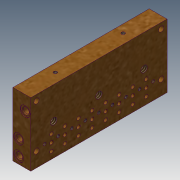
# Autodesk Inventor part: J005162
Saved by Autodesk Inventor 2015 SP1 (Build 190203100, 203)
## iProperties
Created: 2015-04-08
Material: PEEK 1000
Vendor: HHMI: JRC - ID&F
Document SubType Name: Modeling
Designer: JORDANJ
Density: 1.31 g/cm^3
Appearance: Tan
Project: P-171601
Part Number: J005162
Description: COMPONENT OF AN AUTOMATED LIQUID HANDLING MACHINE SPECIFICALLY DESIGNED FOR THE IN SITU RNA HYBRIDIZATION OF DROSOPHILA EMBRYOS
RuleStatus: InUse
AfterDocSave0: file://Part Number Cleaner
LAB/DEPT: STERN (LAB)
REQUESTING SCIENTIST: STERN, DAVID
SURFACE ROUGHNESS: 16 Ra
DESIGN DEPARTMENT: HHMI: JRC - ID&F
SPECIAL FINISH: N/A
ALTERED ITEM PART NUMBER: N/A
ALTERED ITEM VENDOR: N/A
ALTERED ITEM DESCRIPTION: N/A
valve_spacing: 0.3000 in
no_valves: 8.0000 ul
Author: JORDANJ
Revision Number: A
Autodesk Inventor part; units mm, degrees
ref_plane "YZ Plane" through (0, 0, 0) normal (1, 0, 0) x (0, 1, 0)
ref_plane "XZ Plane" through (0, 0, 0) normal (0, 1, 0) x (-1, 0, 0)
ref_plane "XY Plane" through (0, 0, 0) normal (0, 0, 1) x (1, 0, 0)
sketch "Sketch1" plane through (0, 0, 0) normal (0, 0, 1) x (1, 0, 0)
  line L0 (9.9949, 17.907) -> (0, 17.907)
  line L1 (0, 17.907) -> (0, -17.907)
  line L2 (0, -17.907) -> (9.9949, -17.907)
  line L3 (9.9949, -17.907) -> (9.9949, 17.907)
  line L4 (3.175, -4.4958) -> (9.9949, -4.4958)
  line L5 (9.9949, -4.4958) -> (9.9949, -6.477)
  line L6 (9.9949, -6.477) -> (3.175, -6.477)
  line L7 (3.175, -6.477) -> (3.175, -4.4958) construction
  line L8 (0.75, -8.7376) -> (9.9949, -8.7376)
  line L9 (9.9949, -8.7376) -> (9.9949, -10.7188)
  line L10 (9.9949, -10.7188) -> (0.75, -10.7188)
  line L11 (0.75, -10.7188) -> (0.75, -8.7376) construction
  line L12 (3.175, -12.9794) -> (9.9949, -12.9794)
  line L13 (9.9949, -12.9794) -> (9.9949, -14.9606)
  line L14 (9.9949, -14.9606) -> (3.175, -14.9606)
  line L15 (3.175, -14.9606) -> (3.175, -12.9794) construction
  line L16 (2.5798, -5.4864) -> (9.9949, -5.4864)
  line L17 (0.1548, -9.7282) -> (9.9949, -9.7282)
  line L18 (2.5798, -13.97) -> (9.9949, -13.97)
  line L19 (5.6958, -7.4168) -> (9.9949, -7.4168)
  line L20 (9.9949, -7.4168) -> (9.9949, -9.6012)
  line L21 (9.9949, -9.6012) -> (5.6958, -9.6012)
  line L22 (5.6958, -9.6012) -> (5.6958, -7.4168) construction
  line L23 (5.6958, -7.4168) -> (5.0395, -8.509)
  line L24 (5.0395, -8.509) -> (5.6958, -9.6012)
  line L25 (5.0395, -8.509) -> (9.9949, -8.509)
  line L26 (9.9949, 17.145) -> (17.6149, 17.145) construction
  line L27 (17.6149, 17.145) -> (17.6149, -8.509) construction
  line L28 (17.6149, -8.509) -> (9.9949, -8.509) construction
  line L29 (9.9949, -8.509) -> (9.9949, 17.145) construction
  line L30 (3.175, -4.4958) -> (2.5798, -5.4864)
  line L31 (2.5798, -5.4864) -> (3.175, -6.477)
  line L32 (0.75, -8.7376) -> (0.1548, -9.7282)
  line L33 (0.1548, -9.7282) -> (0.75, -10.7188)
  line L34 (3.175, -12.9794) -> (2.5798, -13.97)
  line L35 (2.5798, -13.97) -> (3.175, -14.9606)
  circle A0 centre (3.175, -5.4864) radius 1.1811
  line L36 (4.0069, -13.97) -> (5.9881, -13.97) construction
  line L37 (5.9881, -13.97) -> (5.9881, -17.907) construction
  line L38 (5.9881, -17.907) -> (4.0069, -17.907) construction
  line L39 (4.0069, -17.907) -> (4.0069, -13.97) construction
  line L40 (4.0069, -13.97) -> (4.9975, -13.3748) construction
  line L41 (4.9975, -13.3748) -> (5.9881, -13.97) construction
  line L42 (4.9975, -13.3748) -> (4.9975, -17.907) construction
  circle A1 centre (3.175, -5.4864) radius 3.175 construction
  line L43 (0, -7.2282) -> (0.75, -7.2282)
  line L44 (0.75, -7.2282) -> (0.75, -12.2282)
  line L45 (0.75, -12.2282) -> (0, -12.2282)
  line L46 (0, -12.2282) -> (0, -7.2282)
  line L47 (0, -9.7282) -> (0.75, -9.7282)
  circle A2 centre (0.25, -11.7282) radius 0.5
  line L48 (-6.35, 19.431) -> (17.6149, 19.431)
  line L49 (17.6149, 19.431) -> (17.6149, 17.907)
  line L50 (17.6149, 17.907) -> (-6.35, 17.907)
  line L51 (-6.35, 17.907) -> (-6.35, 19.431)
  line L52 (-6.35, 17.907) -> (0, 17.907)
  line L53 (0, 17.907) -> (0, -17.907)
  line L54 (0, -17.907) -> (-6.35, -17.907)
  line L55 (-6.35, -17.907) -> (-6.35, 17.907)
  line L56 (-12.7, -10.9093) -> (0, -10.9093)
  line L57 (0, -10.9093) -> (0, -11.3093)
  line L58 (0, -11.3093) -> (-12.7, -11.3093)
  line L59 (-12.7, -11.3093) -> (-12.7, -10.9093)
  line L60 (-12.7, -8.5471) -> (0, -8.5471)
  line L61 (0, -8.5471) -> (0, -8.1471)
  line L62 (0, -8.1471) -> (-12.7, -8.1471)
  line L63 (-12.7, -8.1471) -> (-12.7, -8.5471)
  line L64 (-12.7, 8.5471) -> (0, 8.5471)
  line L65 (0, 8.5471) -> (0, 8.1471)
  line L66 (0, 8.1471) -> (-12.7, 8.1471)
  line L67 (-12.7, 8.1471) -> (-12.7, 8.5471)
  line L68 (-12.7, 9.7282) -> (0, 9.7282)
  line L69 (-12.7, 10.9093) -> (0, 10.9093)
  line L70 (0, 10.9093) -> (0, 11.3093)
  line L71 (0, 11.3093) -> (-12.7, 11.3093)
  line L72 (-12.7, 11.3093) -> (-12.7, 10.9093)
  circle A3 centre (6.8199, 9.7282) radius 1.1811
  line L73 (0, 12.5857) -> (0.75, 12.5857)
  line L74 (0.75, 12.5857) -> (0.75, 11.7411)
  line L75 (0.75, 11.7411) -> (5.6104, 11.7412)
  line L76 (5.6104, 11.7412) -> (6.8199, 9.7282)
  line L77 (6.8199, 9.7282) -> (0, 9.7282)
  line L78 (0, 6.8707) -> (0.75, 6.8707)
  line L79 (0.75, 6.8707) -> (0.75, 7.7153)
  line L80 (0.75, 7.7153) -> (5.6104, 7.7152)
  line L81 (5.6104, 7.7152) -> (6.8199, 9.7282)
  line L82 (0, 12.5857) -> (0, 6.8707)
  line L83 (-6.35, 0) -> (9.9949, 0) construction
  line L84 (-12.7, -8.5471) -> (-12.7, -10.9093)
  line L85 (-12.7, 10.9093) -> (-12.7, 8.5471)
  line L86 (0, 10.9093) -> (0, 8.5471)
  line L87 (0, -8.5471) -> (0, -10.9093)
  line L88 (-12.7, -9.7282) -> (0, -9.7282)
  circle A4 centre (6.8199, 9.7282) radius 3.175 construction
  circle A5 centre (6.8199, 9.7282) radius 1.5812 construction
  circle A6 centre (3.175, -13.97) radius 1.1811
  line L89 (3.9053, 19.431) -> (6.0896, 19.431)
  line L90 (6.0896, 19.431) -> (6.0896, 13.7614)
  line L91 (6.0896, 13.7614) -> (3.9053, 13.7614) construction
  line L92 (3.9053, 13.7614) -> (3.9053, 19.431)
  line L93 (3.9053, 13.7614) -> (4.9975, 13.1051)
  line L94 (4.9975, 13.1051) -> (6.0896, 13.7614)
  line L95 (2.9147, 20.5994) -> (7.0803, 20.5994)
  line L96 (7.0803, 20.5994) -> (7.0803, 19.431)
  line L97 (7.0803, 19.431) -> (2.9147, 19.431)
  line L98 (2.9147, 19.431) -> (2.9147, 20.5994)
  line L99 (4.9974, 19.431) -> (4.9975, 13.1051)
  line L100 (4.9975, 20.5994) -> (4.9974, 19.431)
  line L101 (3.9053, 14.6685) -> (6.0896, 14.6685)
  line L102 (-3.5011, 2.413) -> (6.35, 2.413)
  line L103 (6.35, 2.413) -> (6.35, -2.413) construction
  line L104 (6.35, -2.413) -> (-3.5011, -2.413)
  line L105 (-3.5011, -2.413) -> (-3.5011, 2.413) construction
  line L106 (6.35, 2.413) -> (7.7999, 0)
  line L107 (7.7999, 0) -> (6.35, -2.413)
  line L108 (-3.5011, 2.413) -> (-6.35, 4.8895)
  line L109 (-6.35, 4.8895) -> (-6.35, -4.8895)
  line L110 (-6.35, -4.8895) -> (-3.5011, -2.413)
  line L111 (-6.35, 0) -> (7.7999, 0)
  line L112 (5.2917, 2.413) -> (5.2917, -2.413) construction
  circle A7 centre (6.8199, 9.7282) radius 1.5
  circle A8 centre (6.8199, 9.7282) radius 2.5
  circle A9 centre (3.175, -5.4864) radius 1.5
  circle A10 centre (3.175, -5.4864) radius 2.5
  circle A11 centre (3.175, -13.97) radius 1.5
  circle A12 centre (3.175, -13.97) radius 2.5
  point P0 (0, 0)
  point P1 (4.9975, 17.907)
  point P2 (0, 0)
  dimension "d2" = 118
  dimension "d3" = 2.1844
  dimension "d4" = 1.9812
  dimension "d5" = 5.461
  dimension "d6" = 1.2192
  dimension "d7" = 3.0226
  dimension "d8" = 4.2992
  dimension "d9" = 118
  dimension "d10" = 7.62
  dimension "d11" = 25.654
  dimension "d12" = 0.762
  dimension "d14" = 2.3622
  dimension "d15" = 2.9464
  dimension "d17" = 1
  dimension "d20" = 3
  dimension "d21" = 1.524
  dimension "d22" = 9.398
  dimension "d26" = 6.35
  dimension "port_depth" = 6.35
  dimension "d29" = 118
  dimension "d30" = 4.0259
  dimension "d32" = 5.715
  dimension "d35" = 0.75
  dimension "d36" = 8.1788
  dimension "d38" = 9.9949
  dimension "d45" = 6.35
  dimension "port_id" = 2.3622
  dimension "port_od" = 3.1623
  dimension "d101" = 8.1788
  dimension "d102" = 3.1623
  dimension "d104" = 5.6388
  dimension "d107" = 3.1623
  dimension "d134" = 118
  dimension "d137" = 2.1844
  dimension "d138" = 1.1684
  dimension "d139" = 4.1656
  dimension "drilldepth" = 4.1456
  dimension "d158" = 4.7625
  dimension "d159" = 0.9071
  dimension "threaddepth" = 3.2385
  dimension "d161" = 118
  dimension "d162" = 82
  dimension "d163" = 9.779
  dimension "d164" = 4.826
  dimension "d165" = 12.7
  dimension "d166" = 5.2917
  dimension "d183" = 0.25
  dimension "d212" = 1
  dimension "d213" = 3
  dimension "d284" = 6.35
  dimension "d296" = 0.75
  constraints: 226 end point, 33 parallel, 27 collinear, 22 horizontal, 22 midpoint, 15 perpendicular, 13 equal length, 12 centre point, 12 vertical, 8 coincident, 8 symmetric about line, 6 equal radius, 5 point on line, 3 tangent, 1 vertical alignment, 9 other
  measures "d2" angle of L24 L23
  measures "d3" distance between parallel lines of L21 L19
  measures "d4" distance between parallel lines of L14 L12
  measures "d5" distance between parallel lines of L25 L18
  measures "d6" distance between parallel lines of L17 L25
  measures "d7" distance between parallel lines of L16 L25
  measures "d8" distance of L19.start L19.end
  measures "d9" angle of L41 L40
  measures "d10" distance of L26.start L26.end
  measures "d11" distance of L26.end L27.end
  measures "d12" distance between parallel lines of L26 L0
  measures "d14" diameter of A0
  measures "d15" distance between parallel lines of L38 L14
  measures "d17" diameter of A2
  measures "d21" distance of L48.end L49.end
  measures "d22" distance between parallel lines of L2 L28
  measures "d26" distance between parallel lines of L55 L59
  measures "port_depth" distance between parallel lines of L57 L55
  measures "d29" angle of L81 L76
  measures "d30" distance between parallel lines of L80 L75
  measures "d32" distance of L73.start L78.start
  measures "d35" distance between parallel lines of L82 L79
  measures "d36" distance between parallel lines of L52 L68
  measures "d38" distance of L1.end L2.end
  measures "d45" distance of L53.end L54.end
  measures "port_id" distance between parallel lines of L60 L56
  measures "port_od" distance between parallel lines of L58 L62
  measures "d101" distance between parallel lines of L54 L88
  measures "d102" distance between parallel lines of L71 L66
  measures "d104" distance edge to line of A3 L82
  measures "d107" diameter of A5
  measures "d134" angle of L94 L93
  measures "d137" distance between parallel lines of L90 L92
  measures "d138" distance of L97.end L95.start
  measures "d139" distance between parallel lines of L96 L98
  measures "drilldepth" distance between parallel lines of L91 L0
  measures "d158" distance between parallel lines of L97 L101
  measures "d159" distance between parallel lines of L101 L91
  measures "threaddepth" distance between parallel lines of L101 L0
  measures "d161" angle of L107 L106
  measures "d162" angle of L110 L108
  measures "d163" distance of L108.end L109.end
  measures "d164" distance between parallel lines of L104 L102
  measures "d165" distance between parallel lines of L103 L109
  measures "d166" distance between parallel lines of L112 L1
  measures "d183" distance centre to line of A2 L1
  measures "d212" radial gap between concentric circles of A8 A7
  measures "d213" diameter of A7
  measures "d284" diameter of A4
  measures "d296" distance of L44.end L45.end
sketch "Sketch2" plane through (0, 0, 0) normal (1, 0, 0) x (0, 1, 0)
  line L0 (17.907, 11.6205) -> (-17.907, 11.6205)
  line L1 (-17.907, 11.6205) -> (-17.907, -64.9605)
  line L2 (-17.907, -64.9605) -> (17.907, -64.9605)
  line L3 (17.907, -64.9605) -> (17.907, 11.6205)
  circle A0 centre (-13.97, 0) radius 0.9906 construction
  circle A1 centre (-9.7282, 0) radius 0.9906 construction
  circle A2 centre (-5.4864, 0) radius 1.5812 construction
  line L4 (-8.509, 3.81) -> (-8.509, -3.81) construction
  circle A3 centre (9.7282, 0) radius 1.5812 construction
  circle A4 centre (-8.509, -3.81) radius 2.3876 construction
  circle A5 centre (-8.509, 3.81) radius 2.3876 construction
  line L5 (17.145, 3.81) -> (-17.907, 3.81) construction
  line L6 (-17.907, 3.81) -> (-17.907, -3.81) construction
  line L7 (-17.907, -3.81) -> (17.145, -3.81) construction
  line L8 (17.145, -3.81) -> (17.145, 3.81) construction
  line L9 (17.145, 0) -> (-17.907, 0) construction
  line L10 (24.257, 1.5875) -> (17.145, 1.5875) construction
  line L11 (17.145, 1.5875) -> (17.145, 0.9525) construction
  line L12 (17.145, 0.9525) -> (24.257, 0.9525) construction
  line L13 (24.257, 0.9525) -> (24.257, 1.5875) construction
  line L14 (24.257, -1.5875) -> (17.145, -1.5875) construction
  line L15 (17.145, -1.5875) -> (17.145, -0.9525) construction
  line L16 (17.145, -0.9525) -> (24.257, -0.9525) construction
  line L17 (24.257, -0.9525) -> (24.257, -1.5875) construction
  line L18 (24.257, 1.27) -> (17.145, 1.27) construction
  line L19 (24.257, -1.27) -> (17.145, -1.27) construction
  line L20 (17.907, -26.67) -> (-17.907, -26.67) construction
  line L21 (-8.509, -3.81) -> (-8.509, -11.43) construction
  circle A6 centre (-8.509, -11.43) radius 2.3876 construction
  line L22 (-8.509, -11.43) -> (-8.509, -19.05) construction
  circle A7 centre (-8.509, -19.05) radius 2.3876 construction
  line L23 (-8.509, -19.05) -> (-8.509, -26.67) construction
  circle A8 centre (-8.509, -26.67) radius 2.3876 construction
  line L24 (-8.509, -26.67) -> (-8.509, -34.29) construction
  circle A9 centre (-8.509, -34.29) radius 2.3876 construction
  line L25 (-8.509, -34.29) -> (-8.509, -41.91) construction
  circle A10 centre (-8.509, -41.91) radius 2.3876 construction
  line L26 (-8.509, -41.91) -> (-8.509, -49.53) construction
  circle A11 centre (-8.509, -49.53) radius 2.3876 construction
  line L27 (-8.509, -49.53) -> (-8.509, -57.15) construction
  circle A12 centre (-8.509, -57.15) radius 2.3876 construction
  circle A13 centre (14.6685, 8.382) radius 1.4224
  circle A14 centre (-9.7282, 8.382) radius 1.4224
  circle A15 centre (14.6685, 8.382) radius 2.8575
  circle A16 centre (14.6685, 8.382) radius 3.2385 construction
  line L28 (0, -64.9605) -> (0, 11.6205) construction
  circle A17 centre (14.6685, -61.722) radius 1.4224
  circle A18 centre (-9.7282, -61.722) radius 1.4224
  line L29 (-9.7282, 6.1976) -> (14.6685, 6.1976)
  line L30 (16.8529, 8.382) -> (16.8529, 14.859)
  line L31 (14.6685, 17.0434) -> (-9.7282, 17.0434)
  line L32 (-11.9126, 14.859) -> (-11.9126, 8.382)
  arc A19 (-11.9126, 8.382) -> (-9.7282, 6.1976) centre (-9.7282, 8.382) ccw
  arc A20 (-9.7282, 17.0434) -> (-11.9126, 14.859) centre (-9.7282, 14.859) ccw
  arc A21 (16.8529, 14.859) -> (14.6685, 17.0434) centre (14.6685, 14.859) ccw
  arc A22 (14.6685, 6.1976) -> (16.8529, 8.382) centre (14.6685, 8.382) ccw
  circle A23 centre (14.6685, 14.859) radius 1.4224
  circle A24 centre (-9.7282, 14.859) radius 1.4224
  point P0 (0, 0)
  point P1 (-9.7282, 0)
  point P2 (-8.509, 0)
  point P3 (-8.509, 0)
  point P4 (-8.509, 0)
  point P5 (-13.97, 0)
  point P6 (-13.97, 0)
  point P7 (-13.97, 0)
  point P8 (17.907, 0)
  point P9 (17.907, 0)
  point P10 (17.907, 0)
  point P11 (-8.509, 0)
  point P12 (-8.509, -7.62)
  point P13 (-8.509, -15.24)
  point P14 (-8.509, -22.86)
  point P15 (-8.509, -30.48)
  point P16 (-8.509, -38.1)
  point P17 (-8.509, -45.72)
  point P18 (-8.509, -53.34)
  point P19 (-11.9126, 11.6205)
  dimension "d44" = 1.9812
  dimension "valve_spacing" = 7.62
  dimension "d48" = 4.7752
  dimension "d49" = 7.62
  dimension "d51" = 25.654
  dimension "d52" = 0.635
  dimension "d53" = 2.54
  dimension "d54" = 32.766
  dimension "d57" = 7.62
  dimension "d62" = 30.48
  dimension "d103" = 3.1623
  dimension "d245" = 2.8448
  dimension "d249" = 5.715
  dimension "d272" = 24.3967
  dimension "d273" = 0.381
  dimension "d283" = 0.762
  dimension "d293" = 70.104
  dimension "d294" = 24.3967
  dimension "d295" = 76.581
  constraints: 67 end point, 25 centre point, 14 coincident, 12 midpoint, 11 tangent, 8 equal radius, 8 parallel, 8 point on circle, 8 symmetric about line, 4 horizontal, 4 perpendicular, 4 point on line, 3 collinear, 3 vertical, 2 concentric, 1 horizontal alignment, 1 vertical alignment, 44 other
  measures "d44" diameter of A0
  measures "valve_spacing" distance of L4.start L4.end
  measures "d48" diameter of A4
  measures "d49" distance of L5.end L6.end
  measures "d51" distance between parallel lines of L8 L4
  measures "d52" distance between parallel lines of L12 L10
  measures "d53" distance between parallel lines of L19 L18
  measures "d54" distance between parallel lines of L13 L4
  measures "d57" distance of L4.start L21.start
  measures "d62" distance from line of L20 A5.centre
  measures "d103" diameter of A2
  measures "d245" diameter of A13
  measures "d249" diameter of A15
  measures "d272" distance of A14.centre A13.centre
  measures "d273" radial gap between concentric circles of A16 A15
  measures "d283" radial gap between concentric circles of A22 A13
  measures "d293" distance of A17.centre A13.centre
  measures "d294" distance of A18.centre A17.centre
  measures "d295" distance of A17.centre A23.centre
extrude "Extrusion1" add sketch "Sketch2" along normal blind 9.9949 contours L3 L2 L1 L0 L32 A19 L29 A15 L30 | L30 A15 L29 A19 L32 L0 | L30 A22 L29 A15 | A15 L29 A22 L30
extrude "Extrusion2" add sketch "Sketch2" against normal blind 6.35 separate body contours L3 L2 L1 L0 L32 A19 L29 A15 L30 | L30 A15 L29 A19 L32 L0 | L30 A22 L29 A15 | A15 L29 A22 L30
revolve "Revolution3" cut sketch "Sketch1" angle 360 about axis through (2.5798, -13.97, 0) along (1, 0, 0) bodies 2 1 contours L3 L14 A12 L18 | A12 L14 A11 L18 | A11 L14 A6 L18 | A6 L14 L35 L18
revolve "Revolution4" cut sketch "Sketch1" angle 360 about axis through (0.1548, -9.7282, 0) along (1, 0, 0) bodies 1 contours L3 L10 L44 L17 | L44 L33 L17
revolve "Revolution5" cut sketch "Sketch1" angle 360 about axis through (2.5798, -5.4864, 0) along (1, 0, 0) bodies 1 contours L3 L6 A10 L16 | A10 L6 A9 L16 | A9 L6 A0 L16 | A0 L6 L31 L16
revolve "Revolution6" cut sketch "Sketch1" angle 360 about axis through (0, -9.7282, 0) along (1, 0, 0) bodies 1 contours L44 L33 L17 | L33 L44 A2 L1 L47 | A2 L1 | L44 L45 A2 | L45 L1 A2
revolve "Revolution7" cut sketch "Sketch1" angle 360 about axis through (6.8199, 9.7282, 0) along (-1, 0, 0) bodies 1 contours L77 A8 L80 L79 L78 L1 | L77 A7 L81 L80 A8 | L77 A3 L81 A7 | L77 L81 A3
revolve "Revolution8" cut sketch "Sketch1" angle 360 about axis through (-12.7, 9.7282, 0) along (1, 0, 0) bodies 2 contours L1 L64 L55 L68 | L55 L64 L85 L68 | L1 L66 L55 L64 | L55 L66 L67 L64
revolve "Revolution9" cut sketch "Sketch1" angle 360 about axis through (-12.7, -9.7282, 0) along (1, 0, 0) picked at (-0.0128, -11.3077) bodies 2 contours L1 L56 L55 L88 | L1 A2 L58 L55 L56 | L55 L56 L84 L88 | L1 L58 A2 | L55 L58 L59 L56
sketch "Sketch3" plane through (9.9949, 0, 0) normal (1, 0, 0) x (0, 0, -1)
  circle A0 centre (-3.81, -8.509) radius 2.3876 construction
  circle A1 centre (3.81, -8.509) radius 2.3876 construction
  line L0 (-11.6205, 17.907) -> (-11.6205, -17.907) projected
  line L1 (-11.6205, -17.907) -> (64.9605, -17.907) projected
  line L2 (64.9605, -17.907) -> (64.9605, 17.907) projected
  line L3 (64.9605, 17.907) -> (-11.6205, 17.907) projected
  point P0 (0, 0)
hole "Hole1" at (9.9949, -8.509, 3.81) at (9.9949, -8.509, -3.81) direction (-1, 0, 0) diameter 1.7018 depth 4.2991 tip angle 118 bodies 1
pattern_linear "Rectangular Pattern2" count 8 spacing 7.62 along (0, 0, -1) of "Revolution3", "Revolution4", "Revolution5", "Revolution6", "Revolution7", "Revolution8", "Revolution9", "Hole1" bodies 1
pattern_linear "Rectangular Pattern3" count 8 spacing 7.62 along (0, 0, -1) of "Revolution3", "Revolution4", "Revolution5", "Revolution6", "Revolution7", "Revolution8", "Revolution9" bodies 2
revolve "Revolution10" add sketch "Sketch1" angle 360 about axis through (-12.7, -9.7282, 0) along (1, 0, 0) separate body picked at (-0.0128, -11.3077) contours L1 A2 L58 L55 L56 | L1 L58 A2 | L55 L58 L59 L56
extrude "Extrusion3" cut sketch "Sketch1" along normal through all both and the other way through all contours A0 L16 L30 L4 | L4 L30 L31 L6 A0 | A0 L6 L31 L16 | L77 L81 A3 | A3 L76 L77 | A3 L81 L76 | A6 L18 L34 L12 | L12 L34 L35 L14 A6 | A6 L14 L35 L18 bodies 1
sketch "Sketch4" plane through (0, -17.907, 11.6205) normal (0, 0, 1) x (1, 0, 0)
  circle A0 centre (3.175, 3.937) radius 1.1811 projected
  circle A1 centre (3.175, 12.4206) radius 1.1811 projected
  circle A2 centre (6.8199, 27.6352) radius 1.1811 projected
  line L0 (0, 0) -> (0, 35.814) projected
  line L1 (0, 0) -> (9.9949, 0) projected
  line L2 (9.9949, 35.814) -> (9.9949, 0) projected
  line L3 (0, 35.814) -> (9.9949, 35.814) projected
hole "Hole3" at (6.8199, 9.7282, 11.6205) at (3.175, -5.4864, 11.6205) at (3.175, -13.97, 11.6205) direction (0, 0, -1) diameter 3.1623 depth 6.35 bodies 1
ref_plane "Work Plane1" through (0, -17.907, -26.67) normal (0, 0, 1) x (1, 0, 0)
mirror "Mirror1" about plane through (0, -17.907, -26.67) normal (0, 0, 1) of "Hole3" bodies 1
revolve "Revolution11" add sketch "Sketch1" angle 360 about axis through (0, -9.7282, 0) along (1, 0, 0) separate body contours A2 L1 | L1 L58 A2 | L1 A2 L58
sketch "Sketch5" plane through (0, 17.907, 11.6205) normal (0, 1, 0) x (1, 0, 0)
  line L0 (-6.35, 68.0085) -> (17.6149, 68.0085)
  line L1 (17.6149, 68.0085) -> (17.6149, 8.5725)
  line L2 (17.6149, 8.5725) -> (-6.35, 8.5725)
  line L3 (15.8369, 12.8905) -> (15.8369, 10.3505) construction
  circle A0 centre (15.8369, 12.8905) radius 0.6604
  circle A1 centre (15.8369, 10.3505) radius 0.6604
  circle A2 centre (15.8369, 10.3505) radius 0.889 construction
  circle A3 centre (15.8369, 12.8905) radius 0.889 construction
  circle A4 centre (13.8049, 11.6205) radius 3.81 construction
  circle A5 centre (15.8369, 10.3505) radius 1.778 construction
  line L4 (-6.35, 8.5725) -> (-6.35, 68.0085)
  line L5 (-6.35, 0) -> (-6.35, 76.581) projected
  line L6 (9.9949, 76.581) -> (9.9949, 0) projected
  point P0 (15.8369, 11.6205)
  point P1 (0, 11.6205)
  point P2 (17.6149, 38.2905)
  point P3 (9.9949, 38.2905)
  dimension "receptacle_hole" = 1.3208
  dimension "receptacle_flange" = 1.778
  dimension "d122" = 2.54
  dimension "d124" = 7.62
  dimension "d274" = 5.842
  constraints: 10 end point, 6 centre point, 4 tangent, 3 horizontal alignment, 3 midpoint, 2 coincident, 2 equal radius, 2 vertical, 1 collinear, 1 horizontal, 1 parallel, 1 perpendicular
  measures "receptacle_hole" diameter of A1
  measures "receptacle_flange" diameter of A2
  measures "d122" distance of L3.start L3.end
  measures "d124" diameter of A4
  measures "d274" distance between parallel lines of L6 L3
extrude "Extrusion4" add sketch "Sketch5" along normal blind 1.524 separate body contours L0 L6 L2 L4 | L0 L1 L2 L6 | A0 | A1
extrude "Extrusion5" cut sketch "Sketch5" along normal through all contours A0 | A1 bodies 5
pattern_linear "Rectangular Pattern4" count 8 spacing 7.62 along (0, 0, -1) of "Extrusion5" bodies 5
sketch "Sketch6" plane through (0, 19.431, 11.6205) normal (0, 1, 0) x (1, 0, 0)
  line L0 (0, 0) -> (0, 76.581) projected
  line L1 (9.9949, 76.581) -> (9.9949, 0) projected
  circle A0 centre (15.8369, 66.2305) radius 0.6604 projected
  circle A1 centre (15.8369, 63.6905) radius 0.6604 projected
  circle A2 centre (15.8369, 58.6105) radius 0.6604 projected
  circle A3 centre (15.8369, 56.0705) radius 0.6604 projected
  circle A4 centre (15.8369, 50.9905) radius 0.6604 projected
  circle A5 centre (15.8369, 48.4505) radius 0.6604 projected
  circle A6 centre (15.8369, 43.3705) radius 0.6604 projected
  circle A7 centre (15.8369, 40.8305) radius 0.6604 projected
  circle A8 centre (15.8369, 35.7505) radius 0.6604 projected
  circle A9 centre (15.8369, 33.2105) radius 0.6604 projected
  circle A10 centre (15.8369, 28.1305) radius 0.6604 projected
  circle A11 centre (15.8369, 25.5905) radius 0.6604 projected
  circle A12 centre (15.8369, 20.5105) radius 0.6604 projected
  circle A13 centre (15.8369, 17.9705) radius 0.6604 projected
  circle A14 centre (15.8369, 12.8905) radius 0.6604 projected
  circle A15 centre (15.8369, 10.3505) radius 0.6604 projected
  line L2 (17.6149, 68.0085) -> (-6.35, 68.0085) projected
  line L3 (-6.35, 8.5725) -> (17.6149, 8.5725) projected
  line L4 (17.6149, 8.5725) -> (17.6149, 68.0085) projected
  line L5 (4.5847, 57.3405) -> (4.5847, 19.2405) construction
  circle A16 centre (4.5847, 57.3405) radius 2.0828
  circle A17 centre (4.5847, 19.2405) radius 2.0828
  line L6 (0, 0) -> (9.9949, 0) projected
  line L7 (0, 76.581) -> (9.9949, 76.581) projected
  line L8 (-6.35, 68.0085) -> (-6.35, 8.5725) projected
  point P0 (0, 11.6205)
  point P1 (4.5847, 38.2905)
  point P2 (0, 38.2905)
  point P3 (4.5847, 73.5457)
  dimension "d141" = 4.1656
  dimension "d142" = 38.1
  constraints: 2 centre point, 2 coincident, 2 end point, 2 midpoint, 1 equal radius, 1 horizontal alignment, 1 vertical, 1 vertical alignment
  measures "d141" diameter of A17
  measures "d142" distance of L5.start L5.end
hole "Hole4" at (4.5847, 19.431, -45.72) at (4.5847, 19.431, -7.62) direction (0, -1, 0) diameter 2.4384 end through all bodies 5 clearance for "Flat Head Machine Screw (82)" size "#2" standard "Ansi Unified Screw Threads"
sketch "Sketch7" plane through (0, 17.907, 11.6205) normal (0, 1, 0) x (1, 0, 0)
  circle A0 centre (4.5847, 57.3405) radius 1.2192 projected
  circle A1 centre (4.5847, 19.2405) radius 1.2192 projected
  circle A2 centre (15.8369, 66.2305) radius 0.6604 projected
  circle A3 centre (15.8369, 63.6905) radius 0.6604 projected
  circle A4 centre (15.8369, 58.6105) radius 0.6604 projected
  circle A5 centre (15.8369, 56.0705) radius 0.6604 projected
  circle A6 centre (15.8369, 50.9905) radius 0.6604 projected
  circle A7 centre (15.8369, 48.4505) radius 0.6604 projected
  circle A8 centre (15.8369, 43.3705) radius 0.6604 projected
  circle A9 centre (15.8369, 40.8305) radius 0.6604 projected
  circle A10 centre (15.8369, 35.7505) radius 0.6604 projected
  circle A11 centre (15.8369, 33.2105) radius 0.6604 projected
  circle A12 centre (15.8369, 28.1305) radius 0.6604 projected
  circle A13 centre (15.8369, 25.5905) radius 0.6604 projected
  circle A14 centre (15.8369, 20.5105) radius 0.6604 projected
  circle A15 centre (15.8369, 17.9705) radius 0.6604 projected
  circle A16 centre (15.8369, 12.8905) radius 0.6604 projected
  circle A17 centre (15.8369, 10.3505) radius 0.6604 projected
  line L0 (-6.35, 68.0085) -> (17.6149, 68.0085) projected
  line L1 (17.6149, 68.0085) -> (17.6149, 8.5725) projected
  line L2 (17.6149, 8.5725) -> (-6.35, 8.5725) projected
  line L3 (-6.35, 8.5725) -> (-6.35, 68.0085) projected
hole "Hole5" at (4.5847, 17.907, -7.62) at (4.5847, 17.907, -45.72) direction (0, -1, 0) diameter 1.9304 depth 4.1456 tip angle 118 bodies 1
sketch "Sketch8" plane through (-6.35, 0, 0) normal (-1, 0, 0) x (0, 0, 1)
  circle A0 centre (-53.34, -9.7282) radius 1.5811 projected
  circle A1 centre (-53.34, 9.7282) radius 1.5811 projected
  circle A2 centre (-45.72, -9.7282) radius 1.5811 projected
  circle A3 centre (-45.72, 9.7282) radius 1.5811 projected
  circle A4 centre (-38.1, -9.7282) radius 1.5811 projected
  circle A5 centre (-38.1, 9.7282) radius 1.5811 projected
  circle A6 centre (-30.48, -9.7282) radius 1.5811 projected
  circle A7 centre (-30.48, 9.7282) radius 1.5811 projected
  circle A8 centre (-22.86, -9.7282) radius 1.5811 projected
  circle A9 centre (-22.86, 9.7282) radius 1.5811 projected
  circle A10 centre (-15.24, -9.7282) radius 1.5811 projected
  circle A11 centre (-15.24, 9.7282) radius 1.5811 projected
  circle A12 centre (-7.62, -9.7282) radius 1.5811 projected
  circle A13 centre (-7.62, 9.7282) radius 1.5811 projected
  circle A14 centre (0, -9.7282) radius 1.5811 projected
  circle A15 centre (0, 9.7282) radius 1.5811 projected
  line L0 (11.6205, -17.907) -> (11.6205, 17.907) projected
  line L1 (11.6205, 17.907) -> (-64.9605, 17.907) projected
  line L2 (-64.9605, 17.907) -> (-64.9605, -17.907) projected
  line L3 (-64.9605, -17.907) -> (11.6205, -17.907) projected
  line L4 (-52.07, 0) -> (-1.27, 0) construction
  circle A16 centre (-52.07, 0) radius 4.5974
  circle A17 centre (-1.27, 0) radius 4.5974
  circle A18 centre (-26.67, 0) radius 4.5974
  point P0 (0, 0)
  point P1 (-26.67, -17.907)
  point P2 (-64.9605, 0)
  dimension "d167" = 50.8
  dimension "d168" = 9.1948
  constraints: 3 centre point, 3 coincident, 3 midpoint, 2 end point, 2 equal radius, 1 horizontal, 1 horizontal alignment, 1 vertical alignment
  measures "d167" distance of L4.start L4.end
  measures "d168" diameter of A16
hole "Hole6" at (-6.35, 0, -52.07) at (-6.35, 0, -1.27) at (-6.35, 0, -26.67) direction (1, 0, 0) diameter 5.1054 end through all countersink diameter 9.779 countersink angle 82 bodies 2 clearance for "Flat Head Machine Screw (82)" size "#10" standard "Ansi Unified Screw Threads"
hole "Hole7" at (-6.35, 0, -52.07) at (-6.35, 0, -1.27) at (-6.35, 0, -26.67) direction (1, 0, 0) diameter 3.683 end through all bodies 1 thread size "10-24 UNC" class "2B" standard "ANSI Unified Screw Threads"
sketch "Sketch11" plane through (-6.35, 0, 0) normal (-1, 0, 0) x (0, 0, 1)
  circle A0 centre (-1.27, 0) radius 4.8895 projected
  circle A1 centre (-52.07, 0) radius 4.8895 projected
  circle A2 centre (-26.67, 0) radius 4.8895 projected
  circle A3 centre (-53.34, -9.7282) radius 1.5811 projected
  circle A4 centre (-53.34, 9.7282) radius 1.5811 projected
  circle A5 centre (-45.72, -9.7282) radius 1.5811 projected
  circle A6 centre (-45.72, 9.7282) radius 1.5811 projected
  circle A7 centre (-38.1, -9.7282) radius 1.5811 projected
  circle A8 centre (-38.1, 9.7282) radius 1.5811 projected
  circle A9 centre (-30.48, -9.7282) radius 1.5811 projected
  circle A10 centre (-30.48, 9.7282) radius 1.5811 projected
  circle A11 centre (-22.86, -9.7282) radius 1.5811 projected
  circle A12 centre (-22.86, 9.7282) radius 1.5811 projected
  circle A13 centre (-15.24, -9.7282) radius 1.5811 projected
  circle A14 centre (-15.24, 9.7282) radius 1.5811 projected
  circle A15 centre (-7.62, -9.7282) radius 1.5811 projected
  circle A16 centre (-7.62, 9.7282) radius 1.5811 projected
  circle A17 centre (0, -9.7282) radius 1.5811 projected
  circle A18 centre (0, 9.7282) radius 1.5811 projected
  circle A19 centre (8.382, 14.6685) radius 1.4224 projected
  circle A20 centre (-61.722, -9.7282) radius 1.4224 projected
  circle A21 centre (-61.722, 14.6685) radius 1.4224 projected
  circle A22 centre (8.382, -9.7282) radius 1.4224 projected
  line L0 (11.6205, 17.907) -> (-64.9605, 17.907) projected
  line L1 (-64.9605, 17.907) -> (-64.9605, -17.907) projected
  line L2 (-64.9605, -17.907) -> (11.6205, -17.907) projected
  line L3 (11.6205, -17.907) -> (11.6205, 17.907) projected
  point P0 (0, 0)
hole "Hole10" at (-6.35, -9.7282, 8.382) at (-6.35, 14.6685, 8.382) at (-6.35, 14.6685, -61.722) at (-6.35, -9.7282, -61.722) direction (1, 0, 0) diameter 2.9464 end through all countersink diameter 5.715 countersink angle 82 bodies 2 1 clearance for "Flat Head Machine Screw (82)" size "#4" standard "Ansi Unified Screw Threads"
sketch "Sketch10" plane through (9.9949, 0, 0) normal (1, 0, 0) x (0, 0, -1)
  line L0 (64.9605, -17.907) -> (64.9605, 17.907) projected
  circle A0 centre (61.722, 14.6685) radius 1.4732 projected
  circle A1 centre (-8.382, -9.7282) radius 1.4732 projected
  circle A2 centre (-8.382, 14.6685) radius 1.4732 projected
  circle A3 centre (61.722, -9.7282) radius 1.4732 projected
  circle A4 centre (1.27, 0) radius 1.8415 projected
  circle A5 centre (52.07, 0) radius 1.8415 projected
  circle A6 centre (26.67, 0) radius 1.8415 projected
  circle A7 centre (49.53, -8.509) radius 0.8509 projected
  circle A8 centre (34.29, -8.509) radius 0.8509 projected
  circle A9 centre (19.05, -8.509) radius 0.8509 projected
  circle A10 centre (11.43, -8.509) radius 0.8509 projected
  circle A11 centre (26.67, -8.509) radius 0.8509 projected
  circle A12 centre (41.91, -8.509) radius 0.8509 projected
  circle A13 centre (57.15, -8.509) radius 0.8509 projected
  circle A14 centre (-3.81, -8.509) radius 0.8509 projected
  circle A15 centre (3.81, -8.509) radius 0.8509 projected
  line L1 (64.9605, 17.907) -> (-11.6205, 17.907) projected
  line L2 (-11.6205, 17.907) -> (-11.6205, -17.907) projected
  line L3 (-11.6205, -17.907) -> (64.9605, -17.907) projected
  line L4 (64.9605, -17.907) -> (64.9605, 17.907) projected
  circle A16 centre (-8.382, 14.6685) radius 3.2385 construction
  line L5 (-17.0434, 14.6685) -> (-17.0434, -9.7282) projected
  arc A17 (-17.0434, -9.7282) -> (-14.859, -11.9126) centre (-14.859, -9.7282) ccw projected
  line L6 (-14.859, -11.9126) -> (-8.382, -11.9126) projected
  arc A18 (-8.382, -11.9126) -> (-6.1976, -9.7282) centre (-8.382, -9.7282) ccw projected
  line L7 (-6.1976, -9.7282) -> (-6.1976, 14.6685) projected
  arc A19 (-6.1976, 14.6685) -> (-8.382, 16.8529) centre (-8.382, 14.6685) ccw projected
  line L8 (-8.382, 16.8529) -> (-14.859, 16.8529) projected
  arc A20 (-14.859, 16.8529) -> (-17.0434, 14.6685) centre (-14.859, 14.6685) ccw projected
  circle A21 centre (-8.382, -9.7282) radius 1.4732 projected
  circle A22 centre (-8.382, 14.6685) radius 1.4732 projected
  circle A23 centre (-14.859, -9.7282) radius 1.4732
  circle A24 centre (-14.859, 14.6685) radius 1.4732
  constraints: 2 centre point, 2 concentric, 2 equal radius
ref_plane "Work Plane2" through (19.5199, 0, 0) normal (1, 0, 0) x (0, 0, -1)
extrude "Extrusion9" add sketch "Sketch10" along normal up to surface (9.525 mm away) separate body contours L6 A17 L5 A20 L8 L2 | L2 L8 A19 L7 A18 L6
sketch "Sketch12" plane through (0, -17.907, 11.6205) normal (0, 0, 1) x (1, 0, 0)
  circle A0 centre (3.175, 12.4206) radius 1.5812 construction
  circle A1 centre (6.8199, 27.6352) radius 1.5812 construction
  circle A2 centre (3.175, 3.937) radius 1.5812 construction
  line L0 (0, 0) -> (0, 35.814) projected
  line L1 (0, 0) -> (9.9949, 0) projected
  line L2 (9.9949, 35.814) -> (9.9949, 0) projected
  line L3 (0, 35.814) -> (9.9949, 35.814) projected
  circle A3 centre (3.175, 3.937) radius 2.8312
  circle A4 centre (3.175, 12.4206) radius 2.8312
  circle A5 centre (6.8199, 27.6352) radius 2.8312
  circle A6 centre (3.175, 3.937) radius 1.5 construction
  circle A7 centre (3.175, 3.937) radius 2.5 construction
  point P0 (0, 17.907)
  dimension "d285" = 1
  dimension "d286" = 3
  dimension "d287" = 1.25
  constraints: 5 centre point, 2 equal radius
  measures "d285" radial gap between concentric circles of A7 A6
  measures "d286" diameter of A6
  measures "d287" radial gap between concentric circles of A3 A2
extrude "Extrusion10" cut sketch "Sketch12" against normal blind 0.35 contours A3 | A4 | A5 bodies 1
mirror "Mirror3" about plane through (0, -17.907, -26.67) normal (0, 0, 1) of "Extrusion10" bodies 1
chamfer "Chamfer2" distance 0.381 angle 45 6 edges at (3.175, -12.3889, 11.2705) (3.175, -3.9052, 11.2705) (6.8199, 11.3093, 11.2705) (3.175, -12.3889, -64.6105) (3.175, -3.9052, -64.6105) (6.8199, 11.3093, -64.6105)
body "Solid1"
